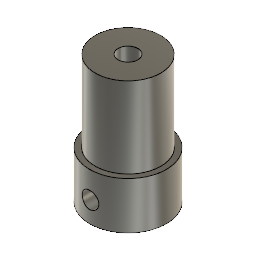
hub v2 (Autodesk Fusion 360 design; units mm, degrees)
Autodesk Fusion 360 part; units mm, degrees
sketch "Sketch1" plane through (0, 0, 0) normal (0, 0, 1) x (1, 0, 0)
  circle A0 centre (0, 0) radius 6.9
  dimension "d1" = 13.8
  constraint coincident A0.centre origin
  measures "d1" diameter of A0
extrude "Extrude1" add sketch "Sketch1" along normal blind 8.5
sketch "Sketch2" plane through (0, 0, 8.5) normal (0, 0, 1) x (-1, 0, 0)
  circle A0 centre (0, 0) radius 6.9
  circle A1 centre (0, 0) radius 5.9
  dimension "d4" = 11.8
  constraint concentric A0 A1
  measures "d4" diameter of A1
extrude "Extrude2" add sketch "Sketch2" along normal blind 14.5 contours A1
sketch "Sketch3" plane through (0, 0, 23) normal (0, 0, 1) x (-1, 0, 0)
  circle A0 centre (0, 0) radius 5.9
  circle A1 centre (0, 0) radius 1.775
  dimension "d7" = 3.55
  constraint coincident A0.centre A1.centre
  measures "d7" diameter of A1
extrude "Extrude3" cut sketch "Sketch3" against normal blind 44 contours A1
sketch "Sketch4" plane through (0, 0, 0) normal (0, 0, -1) x (1, 0, 0)
  circle A0 centre (0, 0) radius 1.775
  circle A1 centre (0, 0) radius 6.9
  circle A2 centre (0, 0) radius 2.1
  dimension "d10" = 4.2
  constraint coincident A0.centre A1.centre
  measures "d10" diameter of A2
extrude "Extrude4" cut sketch "Sketch4" against normal blind 8.5 contours A2
sketch "Sketch5" plane through (0, 0, 0) normal (0, 0, -1) x (1, 0, 0)
  circle A0 centre (0, 0) radius 2.1
  circle A1 centre (0, 0) radius 6.9
  line L0 (0, 0) -> (0, -1.9)
  line L1 (-1.6321, -1.9) -> (0, -1.9)
  line L2 (0, -1.9) -> (1.5021, -1.9)
  constraint coincident A0.centre A1.centre
  constraint vertical L0
  constraint perpendicular L0 L2
extrude "Extrude5" add sketch "Sketch5" against normal blind 8.5 contours A0 L1 L2 picked at (0.1023, -2.0258)
sketch "Sketch6" plane through (0, 1.9, 0) normal (0, -1, 0) x (1, 0, 0)
  line L0 (-0.8944, 0) -> (0.8944, 0)
  line L1 (0.8944, 0) -> (0.8944, 8.5)
  line L2 (0.8944, 8.5) -> (-0.8944, 8.5)
  line L3 (-0.8944, 8.5) -> (-0.8944, 0)
sketch "Sketch7" plane through (0, 0, 0) normal (0, 1, 0) x (1, 0, 0)
  line L0 (-0.5105, -8.5) -> (0.5105, -8.5)
  line L1 (0, 0) -> (0, -7.5)
  circle A0 centre (0, -3.75) radius 1.5
  dimension "d16" = 7.5
  dimension "d17" = 3
  constraint coincident L1.start origin
  constraint perpendicular L0 L1
  constraint midpoint L1 A0.centre
  measures "d16" distance of L1.start L1.end
  measures "d17" diameter of A0
extrude "Extrude6" cut sketch "Sketch7" against normal blind 22
sketch "Sketch8" plane through (0, 0, 0) normal (0, 0, 1) x (1, 0, 0)
  line L0 (0, 0) -> (0, 1.9)
  line L1 (0, 0) -> (0, -0.2117)
  spline S0 degree 3 poles (1.3855, -6.7595) (1.3855, -6.7595) (1.3088, -6.7752) (1.1935, -6.7973) (0.9278, -6.8387) (0.7596, -6.8606) (0.3902, -6.8915) (0.189, -6.9) (-0.189, -6.9) (-0.3902, -6.8915) (-0.7596, -6.8606) (-0.9278, -6.8387) (-1.1935, -6.7973) (-1.3088, -6.7752) (-1.4621, -6.7438) (-1.5, -6.735) (-1.5, -6.735) knots 0 0.056701 0.056701 0.056701 0.056701 0.113401 0.113401 0.170097 0.170097 0.226793 0.226793 0.283489 0.283489 0.340185 0.340185 0.396886 0.396886 0.453586 0.453586 0.453586 0.453586
  circle A0 centre (0, 0) radius 6.9
  line L2 (0, -0.2117) -> (0, -6.9)
  line L3 (0, 0) -> (-6.4839, -2.3599)
  line L4 (0, 0) -> (6.9, 0) construction
  dimension "d20" = 160
  constraint coincident L0.start L1.start
  constraint parallel L0 L1
  constraint coincident A0 L2.end
  constraint parallel L0 L2
  constraint horizontal L4
  constraint coincident A0 L3.end
  measures "d20" angle of L3 L4
ref_plane "WorkPlane1" through (0, 0, 0) normal (-0.939693, -0.34202, 0) x (0.34202, -0.939693, 0)
sketch "Sketch9" plane through (0, 0, 0) normal (-0.939693, -0.34202, 0) x (0.34202, -0.939693, 0)
sketch "Sketch10" plane through (0, 0, 0) normal (-0.939693, -0.34202, 0) x (0.34202, -0.939693, 0)
  line L0 (-1.7854, 0) -> (-1.2717, 0)
  line L1 (0, 0) -> (0, 7.5)
  circle A0 centre (0, 3.75) radius 1.5
  dimension "d22" = 7.5
  dimension "d23" = 3
  constraint coincident L1.start origin
  constraint perpendicular L0 L1
  constraint midpoint L1 A0.centre
  measures "d22" distance of L1.start L1.end
  measures "d23" diameter of A0
extrude "Extrude7" cut sketch "Sketch10" along normal blind 8
extrude "Extrude8" cut 1 faces at (0.9811, 1.7289, 8.5) along direction (0, 0, 1) blind 7
